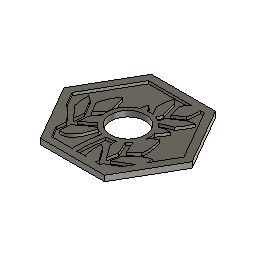
catan_wheat_tile_v1 v2 (Autodesk Fusion 360 design; units mm, degrees)
Autodesk Fusion 360 part; units mm, degrees
note: some values were not read from the file. Chosen so that the rebuilt part matches the saved one: which bodies a step acts on.
sketch "wheat" plane through (0, 0, 0) normal (0, 0, 1) x (1, 0, 0)
  line L0 (-22.805336, 39.5) -> (-45.610671, 0)
  line L1 (-45.610671, 0) -> (-22.805336, -39.5)
  line L2 (-22.805336, -39.5) -> (22.805336, -39.5)
  line L3 (22.805336, -39.5) -> (45.610671, 0)
  line L4 (45.610671, 0) -> (22.805336, 39.5)
  line L5 (22.805336, 39.5) -> (-22.805336, 39.5)
  circle A0 centre (0, 0) radius 12.5
  line L6 (39.837169, 0) -> (19.918584, 34.5)
  line L7 (19.918584, 34.5) -> (-19.918584, 34.5)
  line L8 (-19.918584, 34.5) -> (-39.837169, 0)
  line L9 (-19.918584, -34.5) -> (19.918584, -34.5)
  line L10 (19.918584, -34.5) -> (39.837169, 0)
  line L11 (6.513018, 7.968963) -> (6.516193, 7.968963)
  line L12 (-14.12478, -6.382835) -> (-14.699789, -4.883224)
  line L13 (-14.699789, -4.883224) -> (-14.696614, -4.883224)
  line L14 (11.894114, -4.14906) -> (11.782742, -4.173368)
  line L15 (-10.358587, -11.53038) -> (-10.420315, -11.580359)
  line L16 (5.927867, -15.615467) -> (5.934217, -15.615467)
  line L17 (27.473241, 17.090083) -> (27.469669, 17.090083)
  line L18 (28.131537, -9.4424) -> (28.124393, -9.4424)
  arc A1 (-14.12478, -6.382835) -> (-14.718344, -4.860077) centre (0, 0) ccw
  spline S0 degree 3 poles (28.57193, -29.511966) (28.571926, -29.511968) (28.571923, -29.511969) (28.57192, -29.511971) knots 0.04684767 0.04684767 0.04684767 0.04684767 0.04684874 0.04684874 0.04684874 0.04684874
  spline S1 degree 3 poles (-14.696614, -4.883224) (-14.703849, -4.87551) (-14.711093, -4.867794) (-14.718345, -4.860078) knots 0 0 0 0 0.01380581 0.01380581 0.01380581 0.01380581
  line L19 (-19.918584, -34.5) -> (-39.837169, 0)
  line L20 (7.030699, 29.204885) -> (9.316349, 21.199873)
  line L21 (9.316349, 21.199873) -> (15.935904, 25.668238)
  spline S2 degree 3 poles (0.765133, 32.580344) (-0.384971, 28.506263) (-0.948081, 24.762411) (-0.997143, 21.537994) knots 0 0 0 0 1 1 1 1
  line L22 (-0.997143, 21.537994) -> (2.255113, 15.335073)
  line L23 (5.120829, 14.629666) -> (6.550409, 18.555867)
  line L24 (6.550409, 18.555867) -> (3.432133, 29.456473)
  line L25 (3.432133, 29.456473) -> (3.437488, 29.457417)
  spline S3 degree 3 poles (3.437488, 29.457417) (2.625558, 30.490581) (1.736964, 31.532679) (0.765133, 32.580344) knots 0 0 0 0 1 1 1 1
  line L26 (-57.516356, 13.734317) -> (-57.512009, 13.740972)
  line L27 (-1.61324, 15.415818) -> (-2.896596, 17.861424)
  spline S4 degree 3 poles (-2.896596, 17.861424) (-3.536113, 18.385408) (-4.205271, 18.9084) (-4.909221, 19.427281) knots 0 0 0 0 1 1 1 1
  spline S5 degree 3 poles (21.161409, 23.984118) (20.348436, 23.845921) (19.563066, 23.686828) (18.799977, 23.516205) knots 0 0 0 0 1 1 1 1
  line L28 (18.799977, 23.516205) -> (9.733423, 17.397344)
  line L29 (9.733423, 17.397344) -> (8.191801, 13.158434)
  line L30 (10.054343, 11.796617) -> (17.979258, 15.055656)
  spline S6 degree 3 poles (17.979258, 15.055656) (19.920169, 17.508733) (21.797906, 20.629012) (23.459506, 24.32069) knots 0 0 0 0 1 1 1 1
  spline S7 degree 3 poles (23.459506, 24.32069) (22.674882, 24.222091) (21.906464, 24.11089) (21.161409, 23.984118) knots 0 0 0 0 1 1 1 1
  spline S8 degree 3 poles (-18.917936, 15.312292) (-22.334537, 10.433329) (-24.40099, 5.87948) (-24.977991, 2.161153) knots 0 0 0 0 1 1 1 1
  line L31 (-24.977991, 2.161153) -> (-20.694118, -4.979725)
  line L32 (-20.694118, -4.979725) -> (-15.459781, 1.050105)
  spline S9 degree 3 poles (-15.459781, 1.050105) (-15.273386, 4.893159) (-16.384074, 9.878172) (-18.917936, 15.312292) knots 0 0 0 0 1 1 1 1
  spline S10 degree 3 poles (-31.898327, 3.799839) (-31.954717, -0.430867) (-31.529506, -4.188717) (-30.743526, -7.314477) knots 0 0 0 0 1 1 1 1
  line L33 (-30.743526, -7.314477) -> (-23.304263, -15.38834)
  line L34 (-23.304263, -15.38834) -> (-22.681997, -8.250821)
  line L35 (-22.681997, -8.250821) -> (-28.520335, 1.473972)
  line L36 (-28.520335, 1.473972) -> (-28.51498, 1.474916)
  spline S11 degree 3 poles (-28.51498, 1.474916) (-29.564992, 2.261457) (-30.689903, 3.04068) (-31.898327, 3.799839) knots 0 0 0 0 1 1 1 1
  line L37 (16.110555, 10.620226) -> (12.51497, 9.144699)
  spline S12 degree 3 poles (19.555912, 10.520501) (18.362462, 10.595681) (17.214623, 10.62719) (16.110555, 10.620226) knots 0 0 0 0 1 1 1 1
  line L38 (-19.311728, -8.547819) -> (-19.933931, -15.685692)
  line L39 (-19.933931, -15.685692) -> (-12.08669, -9.703706)
  line L40 (13.052993, -10.231385) -> (16.457043, -17.826453)
  line L41 (16.457043, -17.826453) -> (22.372232, -12.464225)
  spline S13 degree 3 poles (22.372232, -12.464225) (23.014989, -8.672102) (22.507304, -3.590698) (20.636495, 2.107564) knots 0 0 0 0 1 1 1 1
  line L42 (-24.311531, -26.891193) -> (-23.701426, -19.950221)
  line L43 (-23.701426, -19.950221) -> (-31.622423, -11.363196)
  line L44 (6.19876, -18.945332) -> (12.629905, -27.858364)
  line L45 (12.629905, -27.858364) -> (14.095621, -20.842095)
  line L46 (14.095621, -20.842095) -> (10.04631, -11.803459)
  line L47 (9.458516, -10.491419) -> (9.469224, -10.489531)
  line L48 (-11.403834, -13.439965) -> (-20.330178, -20.252742)
  line L49 (-20.330178, -20.252742) -> (-20.993949, -27.806126)
  spline S14 degree 3 poles (30.015592, -12.727141) (28.422964, -13.163286) (26.92746, -13.649296) (25.527427, -14.179934) knots 0 0 0 0 1 1 1 1
  line L50 (25.527427, -14.179934) -> (17.410895, -21.540043)
  line L51 (17.410895, -21.540043) -> (15.942991, -28.544921)
  line L52 (15.942991, -28.544921) -> (25.90509, -22.68204)
  line L53 (11.236811, -34.5) -> (11.689051, -32.337411)
  line L54 (11.689051, -32.337411) -> (4.848494, -22.864236)
  spline S15 degree 3 poles (4.848494, -22.864236) (4.141887, -22.436736) (3.401302, -22.017989) (2.63091, -21.604493) knots 0 0 0 0 1 1 1 1
  line L55 (23.738622, -27.883501) -> (15.002459, -33.029971)
  line L56 (15.002459, -33.029971) -> (14.694874, -34.5)
  line L57 (-15.061798, -3.65954) -> (-19.311728, -8.547819)
  spline S16 degree 3 poles (-8.756874, -12.789337) (-9.673622, -12.987492) (-10.555503, -13.204754) (-11.403834, -13.439965) knots 0.20462852 0.20462852 0.20462852 0.20462852 1 1 1 1
  spline S17 degree 3 poles (-20.993949, -27.806126) (-16.277132, -29.189994) (-10.779694, -24.323051) (-8.164594, -13.175335) knots 0 0 0 0 0.98438829 0.98438829 0.98438829 0.98438829
  spline S18 degree 3 poles (5.919639, -14.325078) (5.920012, -15.97162) (6.015972, -17.516931) (6.19876, -18.945332) knots 0.55315596 0.55315596 0.55315596 0.55315596 1 1 1 1
  spline S19 degree 3 poles (15.052235, 3.698666) (16.595408, 5.496694) (18.119163, 7.764376) (19.555912, 10.520501) knots 0.73674461 0.73674461 0.73674461 0.73674461 1 1 1 1
  spline S20 degree 3 poles (-4.909221, 19.427281) (-5.303808, 17.642738) (-5.566763, 15.968169) (-5.711074, 14.409498) knots 0 0 0 0 0.16042136 0.16042136 0.16042136 0.16042136
  spline S21 degree 3 poles (10.411026, 34.5) (8.909838, 32.670047) (7.772945, 30.887395) (7.030699, 29.204885) knots 0.51122677 0.51122677 0.51122677 0.51122677 1 1 1 1
  spline S22 degree 3 poles (15.935904, 25.668238) (16.702201, 28.058387) (17.059386, 31.061055) (16.925667, 34.5) knots 0 0 0 0 0.65258024 0.65258024 0.65258024 0.65258024
  spline S23 degree 3 poles (-31.622423, -11.363196) (-32.324701, -11.046368) (-33.052824, -10.739691) (-33.809353, -10.440483) knots 0 0 0 0 0.93169949 0.93169949 0.93169949 0.93169949
  spline S24 degree 3 poles (2.63091, -21.604493) (2.218173, -27.099255) (2.846778, -31.434499) (4.142076, -34.5) knots 0 0 0 0 0.48347938 0.48347938 0.48347938 0.48347938
  line L58 (13.052993, -10.231385) -> (12.546525, -9.101358)
  arc A2 (20.636495, 2.107564) -> (15.353761, -2.124153) centre (26.543285, -10.67953) ccw
  line L59 (25.90509, -22.68204) -> (27.17224, -21.936299)
  line L60 (30.015592, -12.727141) -> (30.378043, -16.383686)
  spline S25 degree 3 poles (-3.59106, -15.078272) (-4.67049, -21.403376) (-5.328581, -27.849639) (-5.393314, -34.5) knots 0.26052252 0.26052252 0.26052252 0.26052252 0.67620759 0.67620759 0.67620759 0.67620759
  spline S26 degree 3 poles (-2.007758, -34.5) (-1.944858, -28.008486) (-1.297854, -21.708121) (-0.230315, -15.498289) knots 0.32263192 0.32263192 0.32263192 0.32263192 0.74214201 0.74214201 0.74214201 0.74214201
  dimension "d1" = 39.5
  dimension "d2" = 25
  dimension "d3" = -5
  constraint coincident A0.centre A1.centre
  constraint concentric A0 A1
  constraint parallel L40 L58
  constraint parallel L52 L59
  measures "d1" distance of A0.centre L5
  measures "d2" diameter of A0
extrude "Extrude1" add sketch "wheat" along normal blind 4 contours L0 L1 L2 L3 L4 L5 | L10 S14 L50 L51 L52 L59 L60 | L7 L20 L21 S21 S22 | L9 L10 L55 L56 | L19 L42 L43 S23 | L9 L53 L54 S15 S24 | L9 A1 S25 S26 | L12 L13 A1 S1 L32 S9 | A1 L44 L45 L46 S18 | A1 L48 L49 S16 S17 | A1 L40 L41 S13 L58 A2 | L12 L13 A1 S1 L38 L39 L57 | A1 L37 S12 S19 | A1 S5 L28 L29 L30 S6 S7 | A1 S8 L31 L32 S9 | A1 S2 L22 L23 L24 L25 S3 | A1 L27 S4 S20 | S10 L33 L34 L35 L36 S11 picked at (-0.669253, -37.833333) picked at (22.947804, -19.467339) picked at (10.760984, 25.357665) picked at (19.553222, -31.80449) picked at (-26.545127, -19.401537) picked at (6.362985, -27.303438) picked at (-2.967636, -21.805485) picked at (-14.302466, 2.222693) picked at (10.974762, -22.548597) picked at (-13.912829, -17.564497) picked at (17.29409, -13.507354) picked at (-17.110783, -11.312406) picked at (15.932756, 8.663832) picked at (16.142282, 19.547045) picked at (-20.378962, -0.591407) picked at (3.048947, 24.117844) picked at (-3.767987, 16.642906) picked at (-25.576595, -10.317879) makes body 1 at (20.515472, -33.471157, 0) makes body 1 at (-20.378962, -0.591407, 0) makes body 2 at (-25.576595, -10.317879, 0)
extrude "Extrude2" add sketch "wheat" along normal blind 2 contours L6 L7 L8 L9 L10 A1 L19 L20 L21 S2 L22 L23 L24 L25 S3 L27 S4 S5 L28 L29 L30 S6 S7 S8 L31 L32 S9 L37 S12 L38 L39 L40 L41 S13 L42 L43 L44 L45 L46 L48 L49 S14 L50 L51 L52 L53 L54 S15 L55 L56 L57 S16 S17 S18 S19 S20 S21 S22 S23 S24 L58 A2 L59 L60 S25 S26 picked at (-14.581914, 23.079858) bodies 1 2
sketch "Sketch5" plane through (0, 0, 0) normal (0, 0, 1) x (1, 0, 0)
  spline S0 degree 3 poles (-28.51498, 1.474916) (-29.05141, 1.876744) (-29.59524, 2.267562) (-30.72296, 3.04405) (-31.306468, 3.42802) (-31.898327, 3.799839) knots -0.41074337 -0.41074337 -0.41074337 -0.41074337 -0.20968805 -0.20968805 0 0 0 0
  line L0 (-28.51498, 1.474916) -> (-28.520335, 1.473972)
  line L1 (-28.520335, 1.473972) -> (-22.681997, -8.250821)
  line L2 (-22.681997, -8.250821) -> (-23.304263, -15.38834)
  line L3 (-23.304263, -15.38834) -> (-30.743526, -7.314477)
  spline S1 degree 3 poles (-31.898327, 3.799839) (-31.924828, 1.81157) (-31.846621, -0.196833) (-31.453652, -3.895734) (-31.165584, -5.635996) (-30.743526, -7.314477) knots -1.11396456 -1.11396456 -1.11396456 -1.11396456 -0.51921961 -0.51921961 0 0 0 0
  line L4 (11.236811, -34.5) -> (14.694874, -34.5)
  line L5 (14.694874, -34.5) -> (15.002459, -33.029971)
  line L6 (15.002459, -33.029971) -> (23.738622, -27.883501)
  line L7 (23.738622, -27.883501) -> (27.17224, -21.936299)
  line L8 (27.17224, -21.936299) -> (15.942991, -28.544921)
  line L9 (15.942991, -28.544921) -> (17.410895, -21.540043)
  line L10 (17.410895, -21.540043) -> (25.527427, -14.179934)
  spline S2 degree 3 poles (30.015592, -12.727141) (29.238671, -12.939903) (28.465579, -13.169812) (26.969603, -13.654531) (26.244655, -13.908091) (25.527427, -14.179934) knots -0.47175473 -0.47175473 -0.47175473 -0.47175473 -0.23010503 -0.23010503 0 0 0 0
  line L11 (30.015592, -12.727141) -> (30.378043, -16.383686)
  line L12 (30.378043, -16.383686) -> (39.837169, 0)
  line L13 (39.837169, 0) -> (19.918584, 34.5)
  line L14 (19.918584, 34.5) -> (16.925667, 34.5)
  spline S3 degree 3 poles (15.935904, 25.668238) (16.351085, 26.963226) (16.614177, 28.336749) (16.948756, 31.276399) (16.987779, 32.902614) (16.925667, 34.5) knots -0.88913341 -0.88913341 -0.88913341 -0.88913341 -0.47957782 -0.47957782 0 0 0 0
  line L15 (15.935904, 25.668238) -> (9.316349, 21.199873)
  line L16 (9.316349, 21.199873) -> (7.030699, 29.204885)
  spline S4 degree 3 poles (10.411026, 34.5) (9.705686, 33.640188) (9.034262, 32.734126) (7.909311, 30.971506) (7.425837, 30.100576) (7.030699, 29.204885) knots -0.62698751 -0.62698751 -0.62698751 -0.62698751 -0.29369306 -0.29369306 0 0 0 0
  line L17 (10.411026, 34.5) -> (-19.918584, 34.5)
  line L18 (-19.918584, 34.5) -> (-39.837169, 0)
  line L19 (-39.837169, 0) -> (-33.809353, -10.440483)
  spline S5 degree 3 poles (-31.622423, -11.363196) (-31.978114, -11.202728) (-32.336012, -11.04686) (-33.064996, -10.73942) (-33.436509, -10.587943) (-33.809353, -10.440483) knots -0.2373371 -0.2373371 -0.2373371 -0.2373371 -0.12028356 -0.12028356 0 0 0 0
  line L20 (-31.622423, -11.363196) -> (-23.701426, -19.950221)
  line L21 (-23.701426, -19.950221) -> (-24.311531, -26.891193)
  line L22 (-24.311531, -26.891193) -> (-19.918584, -34.5)
  line L23 (-19.918584, -34.5) -> (-5.393314, -34.5)
  spline S6 degree 3 poles (-3.59106, -15.078272) (-4.134291, -18.261426) (-4.566974, -21.452785) (-5.184014, -27.940329) (-5.361316, -31.212609) (-5.393314, -34.5) knots -1.95481518 -1.95481518 -1.95481518 -1.95481518 -0.98626407 -0.98626407 0 0 0 0
  arc A0 (-8.164593, -13.175334) -> (-3.59106, -15.078272) centre (0, 0) ccw
  spline S7 degree 3 poles (-20.993949, -27.806126) (-20.53089, -27.941983) (-20.056592, -28.018687) (-19.087794, -28.048029) (-18.605108, -27.999234) (-17.173793, -27.679232) (-16.284985, -27.241707) (-14.323467, -25.859629) (-13.200644, -24.675536) (-10.551772, -20.702041) (-9.152438, -17.386344) (-8.164594, -13.175335) knots -3.27669255 -3.27669255 -3.27669255 -3.27669255 -2.99268846 -2.99268846 -2.70622823 -2.70622823 -2.1296213 -2.1296213 -1.29759737 -1.29759737 0 0 0 0
  line L24 (-20.993949, -27.806126) -> (-20.330178, -20.252742)
  line L25 (-20.330178, -20.252742) -> (-11.403834, -13.439965)
  spline S8 degree 3 poles (-8.756874, -12.789337) (-9.207965, -12.88684) (-9.657857, -12.990535) (-10.540191, -13.207538) (-10.97297, -13.320502) (-11.403834, -13.439965) knots -0.27258843 -0.27258843 -0.27258843 -0.27258843 -0.13413575 -0.13413575 0 0 0 0
  arc A1 (-12.08669, -9.703706) -> (-8.756874, -12.789337) centre (0, 0) ccw
  line L26 (-12.08669, -9.703706) -> (-19.933931, -15.685692)
  line L27 (-19.933931, -15.685692) -> (-19.311728, -8.547819)
  line L28 (-19.311728, -8.547819) -> (-15.061798, -3.65954)
  arc A2 (-15.464777, 1.04435) -> (-15.061798, -3.65954) centre (0, 0) ccw
  line L29 (-15.464777, 1.04435) -> (-20.694118, -4.979725)
  line L30 (-20.694118, -4.979725) -> (-24.977991, 2.161153)
  spline S9 degree 3 poles (-18.917936, 15.312292) (-20.457949, 13.113129) (-21.897001, 10.732472) (-23.89796, 6.37304) (-24.654037, 4.248787) (-24.977991, 2.161153) knots -1.43273361 -1.43273361 -1.43273361 -1.43273361 -0.63378591 -0.63378591 0 0 0 0
  spline S10 degree 3 poles (-15.452901, 1.207418) (-15.378289, 3.120125) (-15.619425, 5.302789) (-16.818911, 10.286513) (-17.780846, 12.873687) (-18.917936, 15.312292) knots -1.54502601 -1.54502601 -1.54502601 -1.54502601 -0.80720469 -0.80720469 0 0 0 0
  arc A3 (-5.711074, 14.409498) -> (-15.452901, 1.207418) centre (0, 0) ccw
  spline S11 degree 3 poles (-4.909221, 19.427281) (-5.099098, 18.56855) (-5.265822, 17.702149) (-5.531884, 16.02994) (-5.636052, 15.219795) (-5.711074, 14.409498) knots -0.50791377 -0.50791377 -0.50791377 -0.50791377 -0.24412874 -0.24412874 0 0 0 0
  spline S12 degree 3 poles (-2.896596, 17.861424) (-3.220903, 18.127143) (-3.548, 18.388648) (-4.218912, 18.911223) (-4.562158, 19.171461) (-4.909221, 19.427281) knots -0.25511224 -0.25511224 -0.25511224 -0.25511224 -0.12934724 -0.12934724 0 0 0 0
  line L31 (-2.896596, 17.861424) -> (-1.61324, 15.415818)
  arc A4 (2.255113, 15.335073) -> (-1.61324, 15.415818) centre (0, 0) ccw
  line L32 (2.255113, 15.335073) -> (-0.997143, 21.537994)
  spline S13 degree 3 poles (0.765133, 32.580344) (0.224555, 30.665423) (-0.220164, 28.703649) (-0.798419, 25.026753) (-0.970796, 23.269578) (-0.997143, 21.537994) knots -1.11464932 -1.11464932 -1.11464932 -1.11464932 -0.51953536 -0.51953536 0 0 0 0
  spline S14 degree 3 poles (3.437488, 29.457417) (3.02297, 29.984882) (2.59722, 30.503542) (1.706661, 31.545174) (1.240901, 32.067451) (0.765133, 32.580344) knots -0.41113205 -0.41113205 -0.41113205 -0.41113205 -0.20987443 -0.20987443 0 0 0 0
  line L33 (3.437488, 29.457417) -> (3.432133, 29.456473)
  line L34 (3.432133, 29.456473) -> (6.550409, 18.555867)
  line L35 (6.550409, 18.555867) -> (5.120829, 14.629666)
  arc A5 (8.191801, 13.158434) -> (5.120829, 14.629666) centre (0, 0) ccw
  line L36 (8.191801, 13.158434) -> (9.733423, 17.397344)
  line L37 (9.733423, 17.397344) -> (18.799977, 23.516205)
  spline S15 degree 3 poles (21.161409, 23.984118) (20.760274, 23.915929) (20.36111, 23.841847) (19.573365, 23.684888) (19.186805, 23.602698) (18.799977, 23.516205) knots -0.24104171 -0.24104171 -0.24104171 -0.24104171 -0.11891407 -0.11891407 0 0 0 0
  spline S16 degree 3 poles (23.459506, 24.32069) (23.07136, 24.271914) (22.682732, 24.219495) (21.917222, 24.107715) (21.53842, 24.048266) (21.161409, 23.984118) knots -0.23210022 -0.23210022 -0.23210022 -0.23210022 -0.1147288 -0.1147288 0 0 0 0
  spline S17 degree 3 poles (17.979258, 15.055656) (19.017728, 16.368157) (19.967987, 17.782607) (21.797949, 20.862887) (22.676069, 22.580081) (23.459506, 24.32069) knots -1.07607218 -1.07607218 -1.07607218 -1.07607218 -0.57263812 -0.57263812 0 0 0 0
  line L38 (17.979258, 15.055656) -> (10.054343, 11.796617)
  arc A6 (12.51497, 9.144699) -> (10.054343, 11.796617) centre (0, 0) ccw
  line L39 (12.51497, 9.144699) -> (16.110555, 10.620226)
  spline S18 degree 3 poles (19.555912, 10.520501) (18.971034, 10.557345) (18.385514, 10.584431) (17.236824, 10.61725) (16.673666, 10.623777) (16.110555, 10.620226) knots -0.34474819 -0.34474819 -0.34474819 -0.34474819 -0.16893656 -0.16893656 0 0 0 0
  spline S19 degree 3 poles (15.052235, 3.698666) (15.878231, 4.661075) (16.642615, 5.692617) (18.147156, 7.961503) (18.883769, 9.231125) (19.555912, 10.520501) knots -0.81713899 -0.81713899 -0.81713899 -0.81713899 -0.43621547 -0.43621547 0 0 0 0
  arc A7 (15.353761, -2.124153) -> (15.052238, 3.698666) centre (0, 0) ccw
  arc A8 (20.636495, 2.107564) -> (15.353761, -2.124153) centre (26.543285, -10.67953) ccw
  spline S20 degree 3 poles (22.372232, -12.464225) (22.694044, -10.565607) (22.727448, -8.350393) (22.1395, -3.199751) (21.486256, -0.480706) (20.636495, 2.107564) knots -1.56286905 -1.56286905 -1.56286905 -1.56286905 -0.81725801 -0.81725801 0 0 0 0
  line L40 (22.372232, -12.464225) -> (16.457043, -17.826453)
  line L41 (16.457043, -17.826453) -> (12.546525, -9.101358)
  arc A9 (10.04631, -11.803459) -> (12.546525, -9.101358) centre (0, 0) ccw
  line L42 (10.04631, -11.803459) -> (14.095621, -20.842095)
  line L43 (14.095621, -20.842095) -> (12.629905, -27.858364)
  line L44 (12.629905, -27.858364) -> (6.19876, -18.945332)
  spline S21 degree 3 poles (5.919639, -14.325078) (5.91982, -15.122107) (5.942404, -15.921571) (6.036048, -17.460897) (6.104179, -18.206225) (6.19876, -18.945332) knots -0.46257098 -0.46257098 -0.46257098 -0.46257098 -0.22354028 -0.22354028 0 0 0 0
  arc A10 (-0.230315, -15.498289) -> (5.919639, -14.325078) centre (0, 0) ccw
  spline S22 degree 3 poles (-2.007758, -34.5) (-1.976633, -31.287837) (-1.802213, -28.09156) (-1.193951, -21.7436) (-0.766472, -18.617092) (-0.230315, -15.498289) knots -1.91323872 -1.91323872 -1.91323872 -1.91323872 -0.94936599 -0.94936599 0 0 0 0
  line L45 (-2.007758, -34.5) -> (4.142076, -34.5)
  spline S23 degree 3 poles (2.63091, -21.604493) (2.448227, -24.036552) (2.446345, -26.550377) (2.979153, -30.840877) (3.409035, -32.765158) (4.142076, -34.5) knots -1.29105545 -1.29105545 -1.29105545 -1.29105545 -0.56500641 -0.56500641 0 0 0 0
  spline S24 degree 3 poles (4.848494, -22.864236) (4.490192, -22.647462) (4.127813, -22.435758) (3.388863, -22.016472) (3.01052, -21.808243) (2.63091, -21.604493) knots -0.25485542 -0.25485542 -0.25485542 -0.25485542 -0.12924989 -0.12924989 0 0 0 0
  line L46 (4.848494, -22.864236) -> (11.689051, -32.337411)
  line L47 (11.689051, -32.337411) -> (11.236811, -34.5)
  line L48 (-22.805336, -39.5) -> (22.805336, -39.5)
  line L49 (-45.610671, 0) -> (-22.805336, -39.5)
  line L50 (-22.805336, 39.5) -> (-45.610671, 0)
  line L51 (22.805336, 39.5) -> (-22.805336, 39.5)
  line L52 (45.610671, 0) -> (22.805336, 39.5)
  line L53 (22.805336, -39.5) -> (45.610671, 0)
  circle A11 centre (0, 0) radius 12.5
sketch "Sketch4" plane through (0, 0, 0) normal (0, 0, 1) x (1, 0, 0)
  line L0 (-2.007758, -34.5) -> (4.142076, -34.5)
  line L1 (23.738622, -27.883501) -> (27.17224, -21.936299)
  line L2 (39.837169, 0) -> (19.918584, 34.5)
  line L3 (19.918584, 34.5) -> (16.925667, 34.5)
  line L4 (-19.918584, 34.5) -> (-39.837169, 0)
  line L5 (-22.805336, 39.5) -> (-45.610671, 0)
  line L6 (22.805336, 39.5) -> (-22.805336, 39.5)
  line L7 (-45.610671, 0) -> (-22.805336, -39.5)
  line L8 (-22.805336, -39.5) -> (22.805336, -39.5)
  line L9 (22.805336, -39.5) -> (45.610671, 0)
  line L10 (45.610671, 0) -> (22.805336, 39.5)
  circle A0 centre (0, 0) radius 12.5
  line L11 (30.378043, -16.383686) -> (39.837169, 0)
  line L12 (-39.837169, 0) -> (-33.809353, -10.440483)
  line L13 (-24.311531, -26.891193) -> (-19.918584, -34.5)
  spline S0 degree 3 poles (-8.756874, -12.789337) (-9.207965, -12.88684) (-9.657857, -12.990535) (-10.540191, -13.207538) (-10.97297, -13.320502) (-11.403834, -13.439965) knots -0.27258843 -0.27258843 -0.27258843 -0.27258843 -0.13413575 -0.13413575 0 0 0 0
  arc A1 (-12.08669, -9.703706) -> (-8.756874, -12.789337) centre (0, 0) ccw
  line L14 (-12.08669, -9.703706) -> (-19.933931, -15.685692)
  line L15 (-19.933931, -15.685692) -> (-19.311728, -8.547819)
  line L16 (-19.311728, -8.547819) -> (-15.061798, -3.65954)
  arc A2 (-15.464777, 1.04435) -> (-15.061798, -3.65954) centre (0, 0) ccw
  line L17 (-15.464777, 1.04435) -> (-20.694118, -4.979725)
  line L18 (-20.694118, -4.979725) -> (-24.977991, 2.161153)
  spline S1 degree 3 poles (-18.917936, 15.312292) (-20.457949, 13.113129) (-21.897001, 10.732472) (-23.89796, 6.37304) (-24.654037, 4.248787) (-24.977991, 2.161153) knots -1.43273361 -1.43273361 -1.43273361 -1.43273361 -0.63378591 -0.63378591 0 0 0 0
  spline S2 degree 3 poles (-15.452901, 1.207418) (-15.378289, 3.120125) (-15.619425, 5.302789) (-16.818911, 10.286513) (-17.780846, 12.873687) (-18.917936, 15.312292) knots -1.54502601 -1.54502601 -1.54502601 -1.54502601 -0.80720469 -0.80720469 0 0 0 0
  arc A3 (-5.711074, 14.409498) -> (-15.452901, 1.207418) centre (0, 0) ccw
  spline S3 degree 3 poles (-4.909221, 19.427281) (-5.099098, 18.56855) (-5.265822, 17.702149) (-5.531884, 16.02994) (-5.636052, 15.219795) (-5.711074, 14.409498) knots -0.50791377 -0.50791377 -0.50791377 -0.50791377 -0.24412874 -0.24412874 0 0 0 0
  spline S4 degree 3 poles (-2.896596, 17.861424) (-3.220903, 18.127143) (-3.548, 18.388648) (-4.218912, 18.911223) (-4.562158, 19.171461) (-4.909221, 19.427281) knots -0.25511224 -0.25511224 -0.25511224 -0.25511224 -0.12934724 -0.12934724 0 0 0 0
  line L19 (-2.896596, 17.861424) -> (-1.61324, 15.415818)
  arc A4 (2.255113, 15.335073) -> (-1.61324, 15.415818) centre (0, 0) ccw
  line L20 (2.255113, 15.335073) -> (-0.997143, 21.537994)
  spline S5 degree 3 poles (0.765133, 32.580344) (0.224555, 30.665423) (-0.220164, 28.703649) (-0.798419, 25.026753) (-0.970796, 23.269578) (-0.997143, 21.537994) knots -1.11464932 -1.11464932 -1.11464932 -1.11464932 -0.51953536 -0.51953536 0 0 0 0
  spline S6 degree 3 poles (3.437488, 29.457417) (3.02297, 29.984882) (2.59722, 30.503542) (1.706661, 31.545174) (1.240901, 32.067451) (0.765133, 32.580344) knots -0.41113205 -0.41113205 -0.41113205 -0.41113205 -0.20987443 -0.20987443 0 0 0 0
  line L21 (3.437488, 29.457417) -> (3.432133, 29.456473)
  line L22 (3.432133, 29.456473) -> (6.550409, 18.555867)
  line L23 (6.550409, 18.555867) -> (5.120829, 14.629666)
  arc A5 (8.191801, 13.158434) -> (5.120829, 14.629666) centre (0, 0) ccw
  line L24 (8.191801, 13.158434) -> (9.733423, 17.397344)
  line L25 (9.733423, 17.397344) -> (18.799977, 23.516205)
  spline S7 degree 3 poles (21.161409, 23.984118) (20.760274, 23.915929) (20.36111, 23.841847) (19.573365, 23.684888) (19.186805, 23.602698) (18.799977, 23.516205) knots -0.24104171 -0.24104171 -0.24104171 -0.24104171 -0.11891407 -0.11891407 0 0 0 0
  spline S8 degree 3 poles (23.459506, 24.32069) (23.07136, 24.271914) (22.682732, 24.219495) (21.917222, 24.107715) (21.53842, 24.048266) (21.161409, 23.984118) knots -0.23210022 -0.23210022 -0.23210022 -0.23210022 -0.1147288 -0.1147288 0 0 0 0
  spline S9 degree 3 poles (17.979258, 15.055656) (19.017728, 16.368157) (19.967987, 17.782607) (21.797949, 20.862887) (22.676069, 22.580081) (23.459506, 24.32069) knots -1.07607218 -1.07607218 -1.07607218 -1.07607218 -0.57263812 -0.57263812 0 0 0 0
  line L26 (17.979258, 15.055656) -> (10.054343, 11.796617)
  arc A6 (12.51497, 9.144699) -> (10.054343, 11.796617) centre (0, 0) ccw
  line L27 (12.51497, 9.144699) -> (16.110555, 10.620226)
  spline S10 degree 3 poles (19.555912, 10.520501) (18.971034, 10.557345) (18.385514, 10.584431) (17.236824, 10.61725) (16.673666, 10.623777) (16.110555, 10.620226) knots -0.34474819 -0.34474819 -0.34474819 -0.34474819 -0.16893656 -0.16893656 0 0 0 0
  spline S11 degree 3 poles (15.052235, 3.698666) (15.878231, 4.661075) (16.642615, 5.692617) (18.147156, 7.961503) (18.883769, 9.231125) (19.555912, 10.520501) knots -0.81713899 -0.81713899 -0.81713899 -0.81713899 -0.43621547 -0.43621547 0 0 0 0
  arc A7 (15.353761, -2.124153) -> (15.052238, 3.698666) centre (0, 0) ccw
  arc A8 (20.636495, 2.107564) -> (15.353761, -2.124153) centre (26.543285, -10.67953) ccw
  spline S12 degree 3 poles (22.372232, -12.464225) (22.694044, -10.565607) (22.727448, -8.350393) (22.1395, -3.199751) (21.486256, -0.480706) (20.636495, 2.107564) knots -1.56286905 -1.56286905 -1.56286905 -1.56286905 -0.81725801 -0.81725801 0 0 0 0
  line L28 (22.372232, -12.464225) -> (16.457043, -17.826453)
  line L29 (16.457043, -17.826453) -> (12.546525, -9.101358)
  arc A9 (10.04631, -11.803459) -> (12.546525, -9.101358) centre (0, 0) ccw
  line L30 (10.04631, -11.803459) -> (14.095621, -20.842095)
  line L31 (14.095621, -20.842095) -> (12.629905, -27.858364)
  line L32 (12.629905, -27.858364) -> (6.19876, -18.945332)
  spline S13 degree 3 poles (5.919639, -14.325078) (5.91982, -15.122107) (5.942404, -15.921571) (6.036048, -17.460897) (6.104179, -18.206225) (6.19876, -18.945332) knots -0.46257098 -0.46257098 -0.46257098 -0.46257098 -0.22354028 -0.22354028 0 0 0 0
  arc A10 (-0.230315, -15.498289) -> (5.919639, -14.325078) centre (0, 0) ccw
  spline S14 degree 3 poles (-2.007758, -34.5) (-1.976633, -31.287837) (-1.802213, -28.09156) (-1.193951, -21.7436) (-0.766472, -18.617092) (-0.230315, -15.498289) knots -1.91323872 -1.91323872 -1.91323872 -1.91323872 -0.94936599 -0.94936599 0 0 0 0
  spline S15 degree 3 poles (2.63091, -21.604493) (2.448227, -24.036552) (2.446345, -26.550377) (2.979153, -30.840877) (3.409035, -32.765158) (4.142076, -34.5) knots -1.29105545 -1.29105545 -1.29105545 -1.29105545 -0.56500641 -0.56500641 0 0 0 0
  spline S16 degree 3 poles (4.848494, -22.864236) (4.490192, -22.647462) (4.127813, -22.435758) (3.388863, -22.016472) (3.01052, -21.808243) (2.63091, -21.604493) knots -0.25485542 -0.25485542 -0.25485542 -0.25485542 -0.12924989 -0.12924989 0 0 0 0
  line L33 (4.848494, -22.864236) -> (11.689051, -32.337411)
  line L34 (11.689051, -32.337411) -> (11.236811, -34.5)
  line L35 (11.236811, -34.5) -> (14.694874, -34.5)
  line L36 (14.694874, -34.5) -> (15.002459, -33.029971)
  line L37 (15.002459, -33.029971) -> (23.738622, -27.883501)
  line L38 (27.17224, -21.936299) -> (15.942991, -28.544921)
  line L39 (15.942991, -28.544921) -> (17.410895, -21.540043)
  line L40 (17.410895, -21.540043) -> (25.527427, -14.179934)
  spline S17 degree 3 poles (30.015592, -12.727141) (29.238671, -12.939903) (28.465579, -13.169812) (26.969603, -13.654531) (26.244655, -13.908091) (25.527427, -14.179934) knots -0.47175473 -0.47175473 -0.47175473 -0.47175473 -0.23010503 -0.23010503 0 0 0 0
  line L41 (30.015592, -12.727141) -> (30.378043, -16.383686)
  spline S18 degree 3 poles (15.935904, 25.668238) (16.351085, 26.963226) (16.614177, 28.336749) (16.948756, 31.276399) (16.987779, 32.902614) (16.925667, 34.5) knots -0.88913341 -0.88913341 -0.88913341 -0.88913341 -0.47957782 -0.47957782 0 0 0 0
  line L42 (15.935904, 25.668238) -> (9.316349, 21.199873)
  line L43 (9.316349, 21.199873) -> (7.030699, 29.204885)
  spline S19 degree 3 poles (10.411026, 34.5) (9.705686, 33.640188) (9.034262, 32.734126) (7.909311, 30.971506) (7.425837, 30.100576) (7.030699, 29.204885) knots -0.62698751 -0.62698751 -0.62698751 -0.62698751 -0.29369306 -0.29369306 0 0 0 0
  line L44 (10.411026, 34.5) -> (-19.918584, 34.5)
  spline S20 degree 3 poles (-31.622423, -11.363196) (-31.978114, -11.202728) (-32.336012, -11.04686) (-33.064996, -10.73942) (-33.436509, -10.587943) (-33.809353, -10.440483) knots -0.2373371 -0.2373371 -0.2373371 -0.2373371 -0.12028356 -0.12028356 0 0 0 0
  line L45 (-31.622423, -11.363196) -> (-23.701426, -19.950221)
  line L46 (-23.701426, -19.950221) -> (-24.311531, -26.891193)
  line L47 (-19.918584, -34.5) -> (-5.393314, -34.5)
  spline S21 degree 3 poles (-3.59106, -15.078272) (-4.134291, -18.261426) (-4.566974, -21.452785) (-5.184014, -27.940329) (-5.361316, -31.212609) (-5.393314, -34.5) knots -1.95481518 -1.95481518 -1.95481518 -1.95481518 -0.98626407 -0.98626407 0 0 0 0
  arc A11 (-8.164593, -13.175334) -> (-3.59106, -15.078272) centre (0, 0) ccw
  spline S22 degree 3 poles (-20.993949, -27.806126) (-20.53089, -27.941983) (-20.056592, -28.018687) (-19.087794, -28.048029) (-18.605108, -27.999234) (-17.173793, -27.679232) (-16.284985, -27.241707) (-14.323467, -25.859629) (-13.200644, -24.675536) (-10.551772, -20.702041) (-9.152438, -17.386344) (-8.164594, -13.175335) knots -3.27669255 -3.27669255 -3.27669255 -3.27669255 -2.99268846 -2.99268846 -2.70622823 -2.70622823 -2.1296213 -2.1296213 -1.29759737 -1.29759737 0 0 0 0
  line L48 (-20.993949, -27.806126) -> (-20.330178, -20.252742)
  line L49 (-20.330178, -20.252742) -> (-11.403834, -13.439965)
  spline S23 degree 3 poles (-28.51498, 1.474916) (-29.05141, 1.876744) (-29.59524, 2.267562) (-30.72296, 3.04405) (-31.306468, 3.42802) (-31.898327, 3.799839) knots -0.41074337 -0.41074337 -0.41074337 -0.41074337 -0.20968805 -0.20968805 0 0 0 0
  line L50 (-28.51498, 1.474916) -> (-28.520335, 1.473972)
  line L51 (-28.520335, 1.473972) -> (-22.681997, -8.250821)
  line L52 (-22.681997, -8.250821) -> (-23.304263, -15.38834)
  line L53 (-23.304263, -15.38834) -> (-30.743526, -7.314477)
  spline S24 degree 3 poles (-31.898327, 3.799839) (-31.924828, 1.81157) (-31.846621, -0.196833) (-31.453652, -3.895734) (-31.165584, -5.635996) (-30.743526, -7.314477) knots -1.11396456 -1.11396456 -1.11396456 -1.11396456 -0.51921961 -0.51921961 0 0 0 0
equation "d1 = ( 79 / 2 ) * 1 mm"
